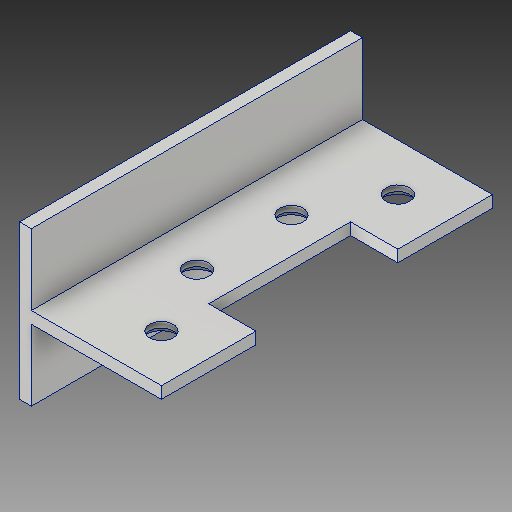
# Autodesk Inventor part: t 2 piece
Saved by Autodesk Inventor 2018.3 (Build 223284000, 284)
## iProperties
Created: 2018-02-15
Part Number: t 2 piece
Material: Aluminum 6061
Document SubType Name: Modeling
Designer: Joe
Density: 2.7 g/cm^3
Appearance: Aluminum - Flat
Mass: 52.5496 g
Surface Area: 136.519 cm^2
Volume: 19.4628 cm^3
Author: Joe
Autodesk Inventor part; units mm, degrees
ref_plane "YZ Plane" through (0, 0, 0) normal (1, 0, 0) x (0, 1, 0)
ref_plane "XZ Plane" through (0, 0, 0) normal (0, 1, 0) x (-1, 0, 0)
ref_plane "XY Plane" through (0, 0, 0) normal (0, 0, 1) x (1, 0, 0)
sketch "Sketch1" plane through (0, 0, 0) normal (0, 1, 0) x (-1, 0, 0)
  line L0 (0, 0) -> (38.1, 0)
  line L1 (38.1, 0) -> (38.1, -88.9)
  line L2 (38.1, -88.9) -> (0, -88.9)
  line L3 (0, -25.4) -> (12.7, -25.4)
  line L4 (12.7, -25.4) -> (12.7, -63.5)
  line L5 (12.7, -63.5) -> (0, -63.5)
  line L6 (0, -88.9) -> (0, -63.5)
  line L7 (0, -25.4) -> (0, 0)
  line L8 (38.1, 0) -> (34.925, 0)
  line L9 (34.925, 0) -> (34.925, -88.9)
  line L10 (34.925, -88.9) -> (38.1, -88.9)
  line L11 (38.1, -88.9) -> (38.1, 0)
  point P0 (12.7, -12.7)
  point P1 (22.225, -31.75)
  point P2 (22.225, -57.15)
  point P3 (12.7, -76.2)
  dimension "d0" = 38.1
  dimension "d1" = 88.9
  dimension "d3" = 38.1
  dimension "d4" = 25.4
  dimension "d5" = 12.7
  dimension "d6" = 12.7
  dimension "d7" = 12.7
  dimension "d8" = 12.7
  dimension "d9" = 15.875
  dimension "d10" = 15.875
  dimension "d11" = 31.75
  dimension "d12" = 31.75
  dimension "d13" = 3.175
  dimension "d35" = 12.7
  constraints: 24 end point, 6 parallel, 3 horizontal, 3 perpendicular, 1 point on line
  measures "d0" distance of L1.end L2.end
  measures "d1" distance of L0.end L1.end
  measures "d3" distance of L3.end L4.end
  measures "d4" distance between parallel lines of L0 L3
  measures "d5" distance from line of L0 point (12.7, -12.7)
  measures "d6" distance from line of L7 point (12.7, -12.7)
  measures "d7" distance from line of L6 point (12.7, -76.2)
  measures "d8" distance from line of L5 point (12.7, -76.2)
  measures "d9" distance from line of L1 point (22.225, -31.75)
  measures "d10" distance from line of L1 point (22.225, -57.15)
  measures "d11" distance from line of L0 point (22.225, -31.75)
  measures "d12" distance from line of L2 point (22.225, -57.15)
  measures "d13" distance of L10.end L9.end
  measures "d35" distance between parallel lines of L4 L6
extrude "Extrusion1" add sketch "Sketch1" along normal blind 3.175
hole "Hole1" at (-12.7, 0, -12.7) at (-22.225, 0, -31.75) at (-22.225, 0, -57.15) at (-12.7, 0, -76.2) direction (0, 1, 0) diameter 6.35 depth 3.175 countersink diameter 9.1948 countersink angle 82
extrude "Extrusion2" add sketch "Sketch1" along normal blind 22.225 and the other way blind 19.05 contours L0 L1 L2 L9
thread "Thread1" size "1/4-20 UNC" class "2B" standard "ANSI Unified Screw Threads" full length
thread "Thread2" size "1/4-20 UNC" class "2B" standard "ANSI Unified Screw Threads" full length
thread "Thread3" size "1/4-20 UNC" class "2B" standard "ANSI Unified Screw Threads" full length
thread "Thread4" size "1/4-20 UNC" class "2B" standard "ANSI Unified Screw Threads" full length
equation "\"d9\" = d10"
body "Solid1"
